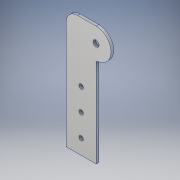
# Autodesk Inventor part: WJ_CLB_027_LifterBracket
Saved by Autodesk Inventor 2018.3 (Build 223284000, 284)
## iProperties
Created: 2020-01-12
Part Number: WJ_CLB_027_LifterBracket
Material: Aluminum 6061
Document SubType Name: Modeling
Designer: 22perngrac
Density: 2.7 g/cm^3
Appearance: Aluminum - Flat
Mass: 23.4019 g
Surface Area: 65.0524 cm^2
Volume: 8.66738 cm^3
Author: 22perngrac
Autodesk Inventor part; units mm, degrees
ref_plane "YZ Plane" through (0, 0, 0) normal (1, 0, 0) x (0, 1, 0)
ref_plane "XZ Plane" through (0, 0, 0) normal (0, 1, 0) x (-1, 0, 0)
ref_plane "XY Plane" through (0, 0, 0) normal (0, 0, 1) x (1, 0, 0)
sketch "Sketch1" plane through (0, 0, 0) normal (0, 0, 1) x (1, 0, 0)
  line L0 (0, 0) -> (25.4, 0)
  line L1 (25.4, 0) -> (25.4, 101.6)
  line L2 (25.4, 101.6) -> (0, 101.6)
  line L3 (0, 101.6) -> (0, 0)
  arc A0 (25.4, 76.2) -> (25.4, 101.6) centre (25.4, 88.9) ccw
  dimension "d0" = 101.6
  dimension "d1" = 25.4
  dimension "d2" = 25.4
  constraints: 8 end point, 2 parallel, 2 point on circle, 2 point on line, 1 centre point, 1 horizontal, 1 perpendicular, 1 tangent
  measures "d0" distance of L2.end L0.start
  measures "d1" distance of L0.start L0.end
  measures "d2" diameter of A0
extrude "Extrusion1" add sketch "Sketch1" along normal blind 2.286
sketch "Sketch3" plane through (0, 0, 2.286) normal (0, 0, 1) x (1, 0, 0)
  line L0 (0, 101.6) -> (0, 0) projected
  line L1 (0, 0) -> (25.4, 0) projected
  line L2 (25.4, 101.6) -> (0, 101.6) projected
  line L3 (25.4, 0) -> (25.4, 76.2) projected
  line L4 (0, 0) -> (25.4, 0)
  line L5 (25.4, 0) -> (25.4, 63.5)
  line L6 (25.4, 63.5) -> (0, 63.5)
  line L7 (0, 63.5) -> (0, 0)
  point P0 (12.7, 50.8)
  point P1 (12.7, 12.7)
  point P2 (12.7, 31.75)
  point P3 (12.7, 0)
  dimension "d50" = 12.7
  dimension "d53" = 38.1
  dimension "d54" = 63.5
  dimension "d55" = 19.05
  constraints: 8 end point, 3 vertical alignment, 2 parallel, 1 horizontal, 1 midpoint, 1 perpendicular, 1 point on line
  measures "d50" distance from line of L1 point (12.7, 12.7)
  measures "d53" distance between parallel lines of L6 L2
  measures "d54" distance between parallel lines of L1 L6
  measures "d55" distance of point (12.7, 12.7) point (12.7, 31.75)
hole "Hole1" at (12.7, 50.8, 2.286) at (12.7, 12.7, 2.286) at (12.7, 31.75, 2.286) direction (0, 0, -1) diameter 3.81 end through all
sketch "Sketch4" plane through (0, 0, 2.286) normal (0, 0, 1) x (1, 0, 0)
  line L0 (25.4, 0) -> (25.4, 76.2) projected
  arc A0 (25.4, 76.2) -> (25.4, 101.6) centre (25.4, 88.9) ccw projected
  point P0 (0, 0)
  constraints: 1 coincident, 1 point on circle
hole "Hole2" at (25.4, 88.9, 2.286) direction (0, 0, -1) diameter 5.08 end through all
fillet "Fillet1" radius 9.525 1 edges at (0, 101.6, 1.143)
fillet "Fillet2" radius 1.5875 1 edges at (25.4, 76.2, 1.143)
equation "\"d2\" = d1"
body "Solid1"
